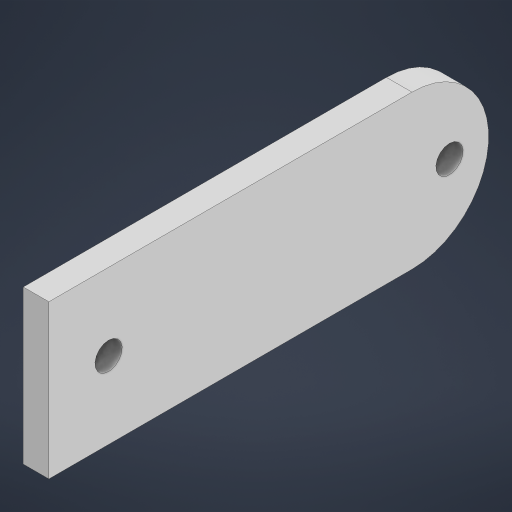
# Autodesk Inventor part: union_servos
Saved by Autodesk Inventor 2023.1 (Build 271208000, 208)
## iProperties
Created: 2022-11-07
Part Number: union_servos
Material: Generic
Document SubType Name: Modeling
Designer: amtat
Density: 1 g/cm^3
Appearance: Default
Author: amtat
Autodesk Inventor part; units mm, degrees
ref_plane "YZ Plane" through (0, 0, 0) normal (1, 0, 0) x (0, 1, 0)
ref_plane "XZ Plane" through (0, 0, 0) normal (0, 1, 0) x (-1, 0, 0)
ref_plane "XY Plane" through (0, 0, 0) normal (0, 0, 1) x (1, 0, 0)
sketch "Sketch1" plane through (0, 0, 0) normal (1, 0, 0) x (0, 1, 0)
  circle A0 centre (0, 0) radius 1.6
  line L0 (0, 0) -> (0, -40)
  circle A1 centre (0, -40) radius 1.6
  line L1 (0, -40) -> (0, -44.6)
  line L2 (0, -44.6) -> (0, -35.6)
  line L3 (0, 0) -> (0, 4.6)
  line L4 (0, 4.6) -> (0, -4.4)
  circle A2 centre (0, -35.6) radius 9
  line L5 (9, -4.4) -> (9, -35.6)
  line L6 (-9, -35.6) -> (-9, -4.4)
  line L7 (0, 0) -> (0, 7)
  line L8 (0, 7) -> (9, 7)
  line L9 (9, 7) -> (9, -4.4)
  line L10 (0, 7) -> (-9, 7)
  line L11 (-9, 7) -> (-9, -4.4)
  dimension "d0" = 3.2
  dimension "d1" = 40
  dimension "d2" = 3.2
  dimension "d3" = 4.6
  dimension "d4" = 9
  dimension "d5" = 4.6
  dimension "d6" = 9
  dimension "d9" = 7
  constraints: 24 end point, 4 point on line, 3 centre point, 3 coincident, 3 perpendicular, 3 point on circle, 3 vertical, 1 tangent
  measures "d0" diameter of A0
  measures "d1" distance of L0.start L0.end
  measures "d2" diameter of A1
  measures "d3" distance of L1.start L1.end
  measures "d4" distance of L1.end L2.end
  measures "d5" distance of L0.start L3.end
  measures "d6" distance of L3.end L4.end
  measures "d9" distance of L0.start L7.end
extrude "Extrusion2" add sketch "Sketch1" along normal blind 3 contours A0 L3 L7 L8 L9 L5 A2 L0 | A0 L0 A2 L6 L11 L10 L7 L3 | A2 L1 A1 L0 | L0 A1 L1 A2
body "Solid2"
